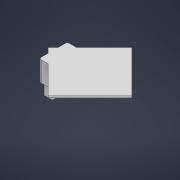
# Autodesk Inventor part: QRholder-top
Saved by Autodesk Inventor 2022 (Build 260153000, 153)
## iProperties
Created: 2023-05-02
Part Number: QRholder-top
Material: Všeobecné
Document SubType Name: Modeling
Designer: tada
Density: 1 g/cm^3
Appearance: Výchozí
Author: tada
Autodesk Inventor part; units mm, degrees
ref_plane "YZ Plane" through (0, 0, 0) normal (1, 0, 0) x (0, 1, 0)
ref_plane "XZ Plane" through (0, 0, 0) normal (0, 1, 0) x (-1, 0, 0)
ref_plane "XY Plane" through (0, 0, 0) normal (0, 0, 1) x (1, 0, 0)
sketch "Náčrt1" plane through (0, 0, 0) normal (0, 1, 0) x (-1, 0, 0)
  line L0 (2.45, 6.925) -> (-2.45, 6.925)
  line L1 (-2.45, 6.925) -> (-2.45, 3.025)
  line L2 (-2.45, 3.025) -> (2.45, 3.025)
  line L3 (2.45, 3.025) -> (2.45, 6.925)
  line L4 (2.45, -3.025) -> (-2.45, -3.025)
  line L5 (-2.45, -3.025) -> (-2.45, -6.925)
  line L6 (-2.45, -6.925) -> (2.45, -6.925)
  line L7 (2.45, -6.925) -> (2.45, -3.025)
  point P0 (0, 0)
  dimension "d0" = 6.05
  dimension "d1" = 3.9
  dimension "d2" = 3.9
  dimension "d3" = 4.9
  dimension "d4" = 4.9
  dimension "d5" = 2.45
  dimension "d6" = 3.025
  constraints: 16 end point, 4 parallel, 2 horizontal, 2 perpendicular, 1 point on line
  measures "d0" distance between parallel lines of L2 L4
  measures "d1" distance between parallel lines of L6 L4
  measures "d2" distance between parallel lines of L0 L2
  measures "d3" distance between parallel lines of L7 L5
  measures "d4" distance between parallel lines of L3 L1
  measures "d5" distance from line of point (0, 0) L7
  measures "d6" distance from line of point (0, 0) L4
extrude "Vysunutí1" add sketch "Náčrt1" along normal blind 7
sketch "Náčrt2" plane through (0, 7, 0) normal (0, 1, 0) x (1, 0, 0)
  line L0 (-3.95, -8.425) -> (3.95, -8.425)
  line L1 (3.95, -8.425) -> (3.95, 8.425)
  line L2 (3.95, 8.425) -> (-3.95, 8.425)
  line L3 (-3.95, 8.425) -> (-3.95, -8.425)
  line L4 (-2.45, -3.025) -> (-2.45, -6.925) projected
  line L5 (-2.45, -6.925) -> (2.45, -6.925) projected
  line L6 (2.45, 6.925) -> (-2.45, 6.925) projected
  line L7 (2.45, 3.025) -> (2.45, 6.925) projected
  point P0 (0, 0)
  dimension "d9" = 1.5
  dimension "d10" = 1.5
  dimension "d11" = 1.5
  dimension "d12" = 1.5
  constraints: 8 end point, 2 parallel, 1 horizontal, 1 perpendicular
  measures "d9" distance between parallel lines of L3 L4
  measures "d10" distance between parallel lines of L0 L5
  measures "d11" distance between parallel lines of L6 L2
  measures "d12" distance between parallel lines of L7 L1
extrude "Vysunutí2" add sketch "Náčrt2" along normal blind 11
sketch "Náčrt3" plane through (0, 18, 0) normal (0, 1, 0) x (1, 0, 0)
  line L0 (-3.95, -8.425) -> (3.95, -8.425) projected
  line L1 (3.95, -8.425) -> (3.95, 8.425) projected
  line L2 (-3.95, 8.425) -> (-3.95, -8.425) projected
  line L3 (-7, 0) -> (18, 25)
  line L4 (18, 25) -> (43, 0)
  line L5 (43, 0) -> (18, -25)
  line L6 (18, -25) -> (-7, 0)
  line L7 (3.95, 8.425) -> (-3.95, 8.425) projected
  line L8 (3.95, 8.425) -> (-3.95, 8.425)
  point P0 (0, 0)
  point P1 (3.95, -8.0855)
  point P2 (3.95, 8.1088)
  point P3 (1.425, -8.425)
  point P4 (1.425, 8.425)
  point P5 (-3.95, 3.05)
  point P6 (-3.95, -3.05)
  dimension "d22" = 90
  dimension "d24" = 90
  dimension "d25" = 135
  dimension "d30" = 7
  dimension "d32" = 0
  dimension "d33" = 25
  dimension "d34" = 25
  dimension "d35" = 3.95
  dimension "d36" = 3.05
  dimension "d40" = 90
  constraints: 10 end point, 1 collinear
  measures "d22" angle of L6 L3
  measures "d24" angle of L3 L4
  measures "d25" angle of L2 L6
  measures "d30" distance of L3.start point (0, 0)
  measures "d32" vertical distance of L3.start point (0, 0)
  measures "d33" horizontal distance of L5.end L3.start
  measures "d34" horizontal distance of L3.start L3.end
  measures "d35" distance from line of L2 point (0, 0)
  measures "d36" distance from line of L3.start L2
  measures "d40" angle of L5 L4
extrude "Vysunutí4" add sketch "Náčrt3" along normal blind 1
fillet "Zaoblení1" radius 1.2 4 edges at (-3.95, 13, 8.425) (3.95, 12.5, 8.425) (3.95, 12.5, -8.425) (-3.95, 13, -8.425)
equation "\"d2\" = d1"
equation "\"d4\" = d3"
equation "\"d5\" = 0.5 * d3"
equation "\"d6\" = 0.5 * d0"
equation "\"d10\" = d9"
equation "\"d11\" = d9"
equation "\"d12\" = d10"
equation "\"d24\" = d22"
